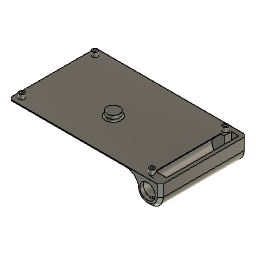
JRCNC0006 v3 (Autodesk Fusion 360 design; units mm, degrees)
Autodesk Fusion 360 part; units mm, degrees
note: some values were not read from the file. Set by a fixed rule: which sketch regions a step uses.
sketch "Sketch1" plane through (0, 0, 0) normal (0, 0, 1) x (1, 0, 0)
  line L0 (0, 0) -> (202, 0)
  line L1 (202, 0) -> (202, 116)
  line L2 (202, 116) -> (0, 116)
  line L3 (0, 116) -> (0, 0)
  dimension "d1" = 202
  dimension "d2" = 116
  constraint horizontal L0
  constraint vertical L1
  constraint horizontal L2
  constraint vertical L3
  constraint coincident L0.start L3.end
  measures "d1" distance of L1.end L2.end
  measures "d2" distance of L0.start L2.end
extrude "Extrude1" add sketch "Sketch1" along normal blind 5
sketch "Sketch2" plane through (0, 0, 0) normal (0, 0, -1) x (-1, 0, 0)
  circle A0 centre (-182, 107) radius 3.5
  line L0 (-182, 107) -> (-182, 9) construction
  line L1 (-182, 9) -> (-8, 9) construction
  circle A1 centre (-182, 9) radius 3.5
  line L2 (-8, 9) -> (-8, 107) construction
  circle A2 centre (-8, 9) radius 3.5
  circle A3 centre (-8, 107) radius 3.5
  line L3 (-8, 107) -> (-182, 107) construction
  line L4 (0, 0) -> (0, 116)
  line L5 (0, 116) -> (-202, 116)
  line L6 (-202, 116) -> (-202, 0)
  line L7 (-202, 0) -> (0, 0)
  dimension "d5" = 174
  dimension "d6" = 98
  dimension "d9" = 7
  dimension "d17" = 8
  dimension "d18" = 9
  constraint horizontal L3
  constraint vertical L0
  constraint horizontal L1
  constraint vertical L2
  constraint coincident L0.end L1.start
  constraint coincident A0.centre L0.start
  constraint coincident L2.end A3.centre
  constraint coincident L1.end L2.start
  constraint equal A2 A3
  constraint equal A1 A3
  constraint equal A0 A3
  measures "d5" distance of L1.end L0.end
  measures "d6" distance of L2.end L1.end
  measures "d9" diameter of A2
  measures "d17" distance of L2 L4
  measures "d18" distance of L1 L7
extrude "Extrude4" add sketch "Sketch2" against normal blind 11 contours A0 | A1 | A2 | A3
sketch "Sketch3" plane through (0, 0, 0) normal (0, -1, 0) x (1, 0, 0)
  line L0 (0, 0) -> (202, 0)
  line L1 (202, 0) -> (202, 5)
  line L2 (202, 5) -> (0, 5)
  line L3 (0, 5) -> (0, 0)
  circle A0 centre (185.5, -10.5) radius 16.5
  line L4 (202, -10.5) -> (202, 5)
  line L5 (169, -10.5) -> (169, 5)
  circle A1 centre (185.5, -10.5) radius 15.5
  dimension "d27" = 33
  dimension "d73" = 31
  constraint coincident A0 L4.start
  constraint coincident L1.end L2.start
  constraint tangent A0 L4
  constraint coincident A0 L5.start
  constraint coincident L2 L5.end
  constraint tangent A0 L5
  constraint perpendicular L2 L5
  constraint vertical L4
  constraint concentric A0 A1
  constraint tangent L2 A1
  measures "d27" diameter of A0
  measures "d73" diameter of A1
extrude "Extrude5" add sketch "Sketch3" against normal blind 116 contours L0 A0 L5 | L0 L2 A0 A1 | L0 A0 A1 | L0 A1 | L0 A1 | L0 A0 L4 | L0 L2 A0 A1
sketch "Sketch4" plane through (0, 0, 0) normal (0, -1, 0) x (1, 0, 0)
  line L0 (0, 0) -> (169, 0)
  line L1 (202, -10.5) -> (202, 5)
  line L2 (202, 5) -> (0, 5)
  line L3 (0, 5) -> (0, 0)
  circle A0 centre (185, -10) radius 10.25
  circle A1 centre (185, -10) radius 14.5
  line L4 (169, 0) -> (169, -10.5)
  arc A2 (169, -10.5) -> (202, -10.5) centre (185.5, -10.5) ccw
  dimension "d30" = 20.5
  dimension "d42" = 29
  constraint concentric A0 A1
  measures "d30" diameter of A0
  measures "d42" diameter of A1
sketch "Sketch5" plane through (0, 0, 5) normal (0, 0, 1) x (-1, 0, 0)
  circle A0 centre (-8, -9) radius 3.5
  circle A1 centre (-8, -107) radius 3.5
  line L0 (0, -116) -> (0, 0)
  line L1 (0, 0) -> (-202, 0)
  line L2 (-202, -116) -> (0, -116)
  line L3 (-197, -13.5) -> (-182, -13.5)
  line L4 (-182, -13.5) -> (-182, -100.5)
  line L5 (-182, -100.5) -> (-197, -100.5)
  line L6 (-197, -100.5) -> (-197, -13.5)
  line L7 (-174.75, 0) -> (-195.25, 0)
  line L8 (-197, -100.5) -> (-187, -100.5)
  line L9 (-187, -100.5) -> (-187, -110)
  line L10 (-187, -110) -> (-197, -110)
  line L11 (-197, -110) -> (-197, -100.5)
  circle A2 centre (-182, -9) radius 3.5
  circle A3 centre (-182, -107) radius 3.5
  line L12 (-202, 0) -> (-202, -116)
  point P0 (-189.5, -100.5)
  dimension "d32" = 87
  dimension "d33" = 13.5
  dimension "d34" = 15
  dimension "d51" = 10
  dimension "d52" = 6
  constraint horizontal L3
  constraint vertical L4
  constraint horizontal L5
  constraint vertical L6
  constraint midpoint L5 P0
  constraint horizontal L8
  constraint vertical L9
  constraint horizontal L10
  constraint vertical L11
  measures "d32" distance of L3.start L5.end
  measures "d33" distance of L3 L7
  measures "d34" distance of L4.end L5.end
  measures "d51" distance of L9.end L10.end
  measures "d52" distance of L2 L10
extrude "Extrude6" cut sketch "Sketch5" against normal blind 20.5 contours L3 L4 L5 L6 L8 | L5 L8 L9 L10 L11
extrude "Extrude7" cut sketch "Sketch4" against normal blind 95.5 from surface at -5 contours A0 | A1
sketch "Sketch6" plane through (0, 13.5, 0) normal (0, 1, 0) x (-1, 0, 0)
  line L0 (-197, 5) -> (-197, -1.8606)
  line L1 (-169, 0) -> (0, 0)
  line L2 (0, 0) -> (0, 5)
  line L3 (0, 5) -> (-202, 5)
  line L4 (-202, 5) -> (-202, -10.5)
  arc A0 (-202, -10.5) -> (-169, -10.5) centre (-185.5, -10.5) ccw
  circle A1 centre (-185.5, -10.5) radius 15
  line L5 (-169, -10.5) -> (-169, 0)
  line L6 (-182, 4.1863) -> (-182, 5)
  arc A2 (-182, 4.1863) -> (-197, -1.8606) centre (-185, -10) ccw
  line L7 (-182, 5) -> (-197, 5)
  dimension "d39" = 30
  constraint concentric A0 A1
  measures "d39" diameter of A1
extrude "Extrude9" cut sketch "Sketch4" against normal blind 33 contours A0
fillet "Fillet2" radius 12.5 1 edges at (169, 58, 0)
sketch "Sketch7" plane through (0, 0, 5) normal (0, 0, 1) x (-1, 0, 0)
  circle A0 centre (-8, -9) radius 3.5
  circle A1 centre (-8, -107) radius 3.5
  line L0 (0, -116) -> (0, 0)
  line L1 (0, 0) -> (-202, 0)
  line L2 (-202, -116) -> (0, -116)
  line L3 (-187, -100.5) -> (-187, -110)
  line L4 (-187, -110) -> (-197, -110)
  line L5 (-197, -110) -> (-197, -100.5)
  line L6 (-197, -13.5) -> (-182, -13.5)
  line L7 (-182, -100.5) -> (-187, -100.5)
  circle A2 centre (-182, -107) radius 3.5
  line L8 (-202, 0) -> (-202, -116)
  line L9 (-182, -13.5) -> (-182, -100.5)
  circle A3 centre (-182, -9) radius 3.5
  line L10 (-197, -100.5) -> (-197, -13.5)
sketch "Sketch8" plane through (0, 0, 5) normal (0, 0, 1) x (-1, 0, 0)
  circle A0 centre (-90, -49.5) radius 8.5
  line L0 (0, -116) -> (0, 0)
  line L1 (0, 0) -> (-202, 0)
  dimension "d53" = 17
  dimension "d54" = 90
  dimension "d55" = 49.5
  measures "d53" diameter of A0
  measures "d54" distance of A0.centre L0
  measures "d55" distance of A0.centre L1
extrude "Extrude10" add sketch "Sketch8" along normal blind 6.4
fillet "Fillet3" radius 2 1 edges at (97.9248, 46.4263, 5)
sketch "Sketch9" plane through (0, 0, 0) normal (0, 0, -1) x (1, 0, 0)
  line L0 (156.569, 0) -> (0, 0)
  line L1 (0, 0) -> (0, -116)
  line L2 (0, -116) -> (156.569, -116)
  line L3 (6.3834, -104.2) -> (4.7668, -107)
  line L4 (4.7668, -107) -> (6.3834, -109.8)
  line L5 (6.3834, -109.8) -> (9.6166, -109.8)
  line L6 (9.6166, -109.8) -> (11.2332, -107)
  line L7 (11.2332, -107) -> (9.6166, -104.2)
  line L8 (9.6166, -104.2) -> (6.3834, -104.2)
  line L9 (6.3834, -6.2) -> (4.7668, -9)
  line L10 (4.7668, -9) -> (6.3834, -11.8)
  line L11 (6.3834, -11.8) -> (9.6166, -11.8)
  line L12 (9.6166, -11.8) -> (11.2332, -9)
  line L13 (11.2332, -9) -> (9.6166, -6.2)
  line L14 (9.6166, -6.2) -> (6.3834, -6.2)
  line L15 (178.7668, -107) -> (180.3834, -109.8)
  line L16 (180.3834, -109.8) -> (183.6166, -109.8)
  line L17 (183.6166, -109.8) -> (185.2332, -107)
  line L18 (185.2332, -107) -> (183.6166, -104.2)
  line L19 (183.6166, -104.2) -> (180.3834, -104.2)
  line L20 (180.3834, -104.2) -> (178.7668, -107)
  line L21 (183.6166, -6.2) -> (180.3834, -6.2)
  line L22 (180.3834, -6.2) -> (178.7668, -9)
  line L23 (178.7668, -9) -> (180.3834, -11.8)
  line L24 (180.3834, -11.8) -> (183.6166, -11.8)
  line L25 (183.6166, -11.8) -> (185.2332, -9)
  line L26 (185.2332, -9) -> (183.6166, -6.2)
  line L27 (156.569, -116) -> (156.569, 0)
  line L28 (156.569, -116) -> (156.569, 0)
  line L29 (156.569, 0) -> (0, 0)
  line L30 (0, 0) -> (0, -116)
  line L31 (0, -116) -> (156.569, -116)
  point P0 (8, -107)
  point P1 (8, -9)
  point P2 (182, -107)
  point P3 (182, -107)
  point P4 (182, -9)
  point P5 (182, -9)
  dimension "d60" = 5.6
  constraint coincident P3 P2
  constraint horizontal L5
  constraint equal L5 L16
  constraint equal L11 L16
  constraint horizontal L14
  constraint horizontal L16
  constraint equal L19 L21
  constraint horizontal L21
  constraint coincident P5 P4
  measures "d60" distance of L5.end L7.end
chamfer "Chamfer3" distance 3 angle 45 2 edges at (0, 116, 2.5) (0, 0, 2.5)
chamfer "Chamfer4" distance 4 angle 45 11 edges at (0, 58, 0) (79.7845, 0, 0) (165.0977, 0, -3.3615) (186.0693, 0, -26.9902) (202, 0, -2.75) (1.5, 1.5, 0) (1.5, 114.5, 0) (79.7845, 116, 0) (165.0977, 116, -3.3615) (186.0693, 116, -26.9902) (202, 116, -2.75)
hole "Hole1" at (182, 9, 0) at (182, 107, 0) at (8, 107, 0) at (8, 9, 0) direction (0, 0, 1) diameter 3.4 end through all
extrude "Extrude11" cut sketch "Sketch9" along normal blind 50 and the other way blind 3.5 contours L3 L4 L5 L6 L7 L8 | L9 L10 L11 L12 L13 L14 | L15 L16 L17 L18 L19 L20 | L21 L22 L23 L24 L25 L26
